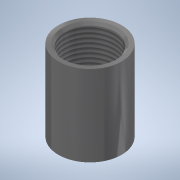
# Autodesk Inventor part: Mufa BSP 1/2'' L=34
Saved by Autodesk Inventor 2020 (Build 240168000, 168)
## iProperties
RuleStatus: InUse
Created: 2022-03-21
Part Number: Mufa BSP 1/2'' L=34
Material: 304
Description: Mufa BSP 1/2'' L=34
Document SubType Name: Modelowanie
Designer: Radosław
Density: 8 g/cm^3
Sheet Metal Rule: 1,5
Sheet Metal Width: 0,000 mm
Sheet Metal Length: 0,000 mm
Sheet Metal Area: 0,000 mm^2
Appearance: Częściowo polerowany(1)
Author: Radosław
Autodesk Inventor part; units mm, degrees
ref_plane "YZ Plane" through (0, 0, 0) normal (1, 0, 0) x (0, 1, 0)
ref_plane "XZ Plane" through (0, 0, 0) normal (0, 1, 0) x (-1, 0, 0)
ref_plane "XY Plane" through (0, 0, 0) normal (0, 0, 1) x (1, 0, 0)
sketch "Szkic5" plane through (0, 0, 0) normal (0, 0, 1) x (1, 0, 0)
  circle A0 centre (0, 0) radius 13.25
  circle A1 centre (0, 0) radius 10.4775
  dimension "d28" = 26.5
  dimension "d29" = 20.955
  constraints: 2 centre point, 2 coincident
  measures "d28" diameter of A0
  measures "d29" diameter of A1
surface extrude "PowWyciągnięciaProstego1" sketch "Szkic5" along normal mid plane 34 shown no curves A0
thicken "Pogrubienie1" operation new thickness 2.7725 both sides no extend neighbours no toward (-0.9870503, 0.1604113, 0) faces at (13.0784, -2.1254, 5.6667)
chamfer "Faza1" distance 1 angle 45 2 edges at (-10.4775, 0, 17) (-10.4775, 0, -17)
thread "Gwint1" size "G20.955x1.814" designation "G 1/2" standard "ISO Pipe Threads" full length
equation "\"d28\" = OD"
equation "\"d29\" = ID"
equation "\"d33\" = L"
equation "\"d35\" = -0.5 * ID + 0.5 * OD"
equation "\"d36\" = OD - 0.5 * ID"
equation "\"SzerokośćGięciaPodcięcia\" = Grubość"
equation "\"RozmiarPodcięciaNarożnika\" = 4 * Grubość"
equation "\"PromieńPrzejścia\" = PromieńGięcia"
equation "\"Rozmiar_promienia_Jacobiego\" = PromieńGięcia"
equation "\"Wielk_odstępu\" = Grubość"
equation "\"d2\" = PromieńGięcia"
equation "\"d23\" = PromieńGięcia"
equation "\"OD\" = 26.5"
equation "\"ID\" = 20.955"
equation "\"L\" = 34"
equation "\"Grubość\" = 1.5"
equation "\"PromieńGięcia\" = 3"
body "Srf1"
